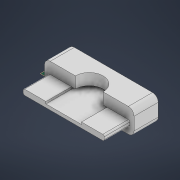
# Autodesk Inventor part: syringe_sledge_fitter
Saved by Autodesk Inventor 2022 (Build 260153000, 153)
## iProperties
Created: 2023-04-24
Part Number: syringe_sledge_fitter
Material: Generic
Document SubType Name: Modeling
Designer: Jakob Saugbjerg
Density: 1 g/cm^3
Appearance: Default
Author: Jakob Saugbjerg
Autodesk Inventor part; units mm, degrees
ref_plane "YZ Plane" through (0, 0, 0) normal (1, 0, 0) x (0, 1, 0)
ref_plane "XZ Plane" through (0, 0, 0) normal (0, 1, 0) x (-1, 0, 0)
ref_plane "XY Plane" through (0, 0, 0) normal (0, 0, 1) x (1, 0, 0)
sketch "Sketch1" plane through (0, 0, 0) normal (0, 0, 1) x (1, 0, 0)
  line L0 (0, 0) -> (63, 0)
  line L1 (63, 0) -> (63, 17)
  line L2 (63, 17) -> (0, 17)
  line L3 (0, 17) -> (0, 0)
  dimension "d0" = 63
  dimension "d1" = 17
  constraints: 8 end point, 2 parallel, 1 horizontal, 1 perpendicular
  measures "d0" distance of L2.end L1.end
  measures "d1" distance of L1.end L0.end
extrude "Extrusion1" add sketch "Sketch1" along normal blind 35
sketch "Sketch2" plane through (0, 17, 0) normal (0, 1, 0) x (1, 0, 0)
  line L0 (31.5, -35) -> (31.5, -17)
  circle A0 centre (31.5, -17) radius 9.75
  line L1 (63, -35) -> (0, -35) projected
  line L2 (21.75, -17) -> (41.25, -17)
  line L3 (41.25, -17) -> (41.25, -35)
  line L4 (41.25, -35) -> (21.75, -35)
  line L5 (21.75, -35) -> (21.75, -17)
  point P0 (0, 0)
  dimension "d37" = 19.5
  dimension "d36" = 18
  constraints: 10 end point, 2 parallel, 1 coincident, 1 horizontal, 1 perpendicular, 1 point on line, 1 vertical, 3 other
  measures "d36" distance of L0.start L0.end
extrude "20 mL cross" cut sketch "Sketch2" against normal blind 8
sketch "Sketch3" plane through (0, 9, 0) normal (0, 1, 0) x (1, 0, 0)
  arc A0 (41.25, -17) -> (21.75, -17) centre (31.5, -17) ccw projected
  circle A1 centre (31.5, -17) radius 12.5
  line L0 (19, -17) -> (44, -17)
  line L1 (44, -17) -> (44, -35)
  line L2 (44, -35) -> (19, -35)
  line L3 (19, -35) -> (19, -17)
  point P0 (0, 0)
  point P1 (41.1047, -25)
  dimension "d40" = 25
  constraints: 8 end point, 2 parallel, 2 point on circle, 1 centre point, 1 coincident, 1 horizontal, 1 perpendicular
  measures "d40" diameter of A1
extrude "20 mL top" cut sketch "Sketch3" against normal blind 1.5
sketch "Sketch4" plane through (0, 17, 0) normal (0, 1, 0) x (1, 0, 0)
  line L0 (63, -35) -> (0, -35)
  line L1 (0, -35) -> (0, -17)
  line L2 (0, -17) -> (63, -17)
  line L3 (63, -17) -> (63, -35)
  point P0 (0, 0)
  dimension "d19" = 63
  dimension "d20" = 18
  constraints: 8 end point, 2 parallel, 1 horizontal, 1 perpendicular
  measures "d19" distance of L1.end L2.end
  measures "d20" distance of L0.end L1.end
extrude "Extrusion4" cut sketch "Sketch4" against normal blind 8
sketch "Sketch10" plane through (0, 0, 0) normal (0, 0, -1) x (-1, 0, 0)
  line L0 (-19.9115, 8.8287) -> (-18.0318, 8.8287)
  line L1 (-18.0318, 8.8287) -> (-18.0318, 8.3965)
  spline S0 degree 2 poles (-18.0318, 8.3965) (-18.2344, 8.2063) (-18.595, 7.8531) (-18.7679, 7.6629) knots 0 0 0 1 2 2 2
  spline S1 degree 2 poles (-18.7679, 7.6629) (-19.1162, 7.28) (-19.3706, 6.8206) (-19.3706, 6.5761) knots 0 0 0 1 2 2 2
  spline S2 degree 2 poles (-19.3706, 6.5761) (-19.3706, 6.4476) (-19.2915, 6.255) (-19.2199, 6.1932) knots 0 0 0 1 2 2 2
  spline S3 degree 2 poles (-19.2199, 6.1932) (-19.1483, 6.1315) (-18.9606, 6.0697) (-18.8469, 6.0697) knots 0 0 0 1 2 2 2
  spline S4 degree 2 poles (-18.8469, 6.0697) (-18.7383, 6.0697) (-18.5159, 6.1241) (-18.4147, 6.1661) knots 0 0 0 1 2 2 2
  spline S5 degree 2 poles (-18.4147, 6.1661) (-18.3282, 6.2006) (-18.1677, 6.2994) (-18.1183, 6.334) knots 0 0 0 1 2 2 2
  line L2 (-18.1183, 6.334) -> (-18.096, 6.334)
  line L3 (-18.096, 6.334) -> (-18.096, 5.8993)
  spline S6 degree 2 poles (-18.096, 5.8993) (-18.222, 5.8375) (-18.674, 5.7165) (-18.8766, 5.7165) knots 0 0 0 1 2 2 2
  spline S7 degree 2 poles (-18.8766, 5.7165) (-19.3039, 5.7165) (-19.7855, 6.1685) (-19.7855, 6.5539) knots 0 0 0 1 2 2 2
  spline S8 degree 2 poles (-19.7855, 6.5539) (-19.7855, 6.7342) (-19.7016, 7.0355) (-19.6275, 7.1639) knots 0 0 0 1 2 2 2
  spline S9 degree 2 poles (-19.6275, 7.1639) (-19.5534, 7.2973) (-19.3385, 7.5591) (-19.2199, 7.6851) knots 0 0 0 1 2 2 2
  spline S10 degree 2 poles (-19.2199, 7.6851) (-19.0272, 7.8951) (-18.5555, 8.3446) (-18.4147, 8.4755) knots 0 0 0 1 2 2 2
  line L4 (-18.4147, 8.4755) -> (-19.9115, 8.4755)
  line L5 (-19.9115, 8.4755) -> (-19.9115, 8.8287)
  spline S11 degree 2 poles (-22.216, 7.3047) (-22.216, 8.1248) (-21.7393, 8.893) (-21.2428, 8.893) knots 0 0 0 1 2 2 2
  spline S12 degree 2 poles (-21.2428, 8.893) (-20.739, 8.893) (-20.2672, 8.11) (-20.2672, 7.3072) knots 0 0 0 1 2 2 2
  spline S13 degree 2 poles (-20.2672, 7.3072) (-20.2672, 6.4822) (-20.7439, 5.719) (-21.2428, 5.719) knots 0 0 0 1 2 2 2
  spline S14 degree 2 poles (-21.2428, 5.719) (-21.7443, 5.719) (-22.216, 6.5094) (-22.216, 7.3047) knots 0 0 0 1 2 2 2
  spline S15 degree 2 poles (-21.6924, 8.2335) (-21.7517, 8.0828) (-21.8011, 7.6184) (-21.8011, 7.3047) knots 0 0 0 1 2 2 2
  spline S16 degree 2 poles (-21.8011, 7.3047) (-21.8011, 6.991) (-21.7517, 6.5292) (-21.6899, 6.3735) knots 0 0 0 1 2 2 2
  spline S17 degree 2 poles (-21.6899, 6.3735) (-21.6282, 6.2179) (-21.4133, 6.0574) (-21.2428, 6.0574) knots 0 0 0 1 2 2 2
  spline S18 degree 2 poles (-21.2428, 6.0574) (-21.0724, 6.0574) (-20.8526, 6.2179) (-20.7884, 6.3785) knots 0 0 0 1 2 2 2
  spline S19 degree 2 poles (-20.7884, 6.3785) (-20.7266, 6.5341) (-20.6822, 7.0083) (-20.6822, 7.3072) knots 0 0 0 1 2 2 2
  spline S20 degree 2 poles (-20.6822, 7.3072) (-20.6822, 7.6283) (-20.7217, 8.0581) (-20.7859, 8.2261) knots 0 0 0 1 2 2 2
  spline S21 degree 2 poles (-20.7859, 8.2261) (-20.8452, 8.3841) (-21.065, 8.5546) (-21.2428, 8.5546) knots 0 0 0 1 2 2 2
  spline S22 degree 2 poles (-21.2428, 8.5546) (-21.4108, 8.5546) (-21.6306, 8.394) (-21.6924, 8.2335) knots 0 0 0 1 2 2 2
  line L6 (-26.5657, 8.8287) -> (-26.5657, 7.5048)
  spline S23 degree 2 poles (-26.5657, 7.5048) (-26.5657, 7.3467) (-26.541, 7.0775) (-26.5015, 7.0034) knots 0 0 0 1 2 2 2
  spline S24 degree 2 poles (-26.5015, 7.0034) (-26.462, 6.9219) (-26.3113, 6.8428) (-26.1804, 6.8428) knots 0 0 0 1 2 2 2
  spline S25 degree 2 poles (-26.1804, 6.8428) (-26.0618, 6.8428) (-25.7901, 6.9886) (-25.6469, 7.1269) knots 0 0 0 1 2 2 2
  spline S26 degree 2 poles (-25.6469, 7.1269) (-25.6494, 7.1615) (-25.6543, 7.2578) (-25.6543, 7.322) knots 0 0 0 1 2 2 2
  line L7 (-25.6543, 7.322) -> (-25.6543, 8.8287)
  line L8 (-25.6543, 8.8287) -> (-25.269, 8.8287)
  line L9 (-25.269, 8.8287) -> (-25.269, 7.5048)
  spline S27 degree 2 poles (-25.269, 7.5048) (-25.269, 7.3467) (-25.2443, 7.0775) (-25.2048, 7.0034) knots 0 0 0 1 2 2 2
  spline S28 degree 2 poles (-25.2048, 7.0034) (-25.1652, 6.9219) (-25.0146, 6.8428) (-24.8837, 6.8428) knots 0 0 0 1 2 2 2
  spline S29 degree 2 poles (-24.8837, 6.8428) (-24.7601, 6.8428) (-24.486, 6.9985) (-24.3575, 7.1195) knots 0 0 0 1 2 2 2
  line L10 (-24.3575, 7.1195) -> (-24.3575, 8.8287)
  line L11 (-24.3575, 8.8287) -> (-23.9722, 8.8287)
  line L12 (-23.9722, 8.8287) -> (-23.9722, 6.5415)
  line L13 (-23.9722, 6.5415) -> (-24.3575, 6.5415)
  line L14 (-24.3575, 6.5415) -> (-24.3575, 6.7934)
  spline S30 degree 2 poles (-24.3575, 6.7934) (-24.5082, 6.6428) (-24.8046, 6.4773) (-24.9825, 6.4773) knots 0 0 0 1 2 2 2
  spline S31 degree 2 poles (-24.9825, 6.4773) (-25.185, 6.4773) (-25.4987, 6.6625) (-25.5802, 6.8725) knots 0 0 0 1 2 2 2
  spline S32 degree 2 poles (-25.5802, 6.8725) (-25.7556, 6.6774) (-26.0865, 6.4773) (-26.2792, 6.4773) knots 0 0 0 1 2 2 2
  spline S33 degree 2 poles (-26.2792, 6.4773) (-26.4274, 6.4773) (-26.6695, 6.5687) (-26.7584, 6.6724) knots 0 0 0 1 2 2 2
  spline S34 degree 2 poles (-26.7584, 6.6724) (-26.8498, 6.7762) (-26.9511, 7.0874) (-26.9511, 7.322) knots 0 0 0 1 2 2 2
  line L15 (-26.9511, 7.322) -> (-26.9511, 8.8287)
  line L16 (-26.9511, 8.8287) -> (-26.5657, 8.8287)
  line L17 (-29.2877, 8.8287) -> (-27.5216, 8.8287)
  line L18 (-27.5216, 8.8287) -> (-27.5216, 5.7807)
  line L19 (-27.5216, 5.7807) -> (-27.9267, 5.7807)
  line L20 (-27.9267, 5.7807) -> (-27.9267, 8.4681)
  line L21 (-27.9267, 8.4681) -> (-29.2877, 8.4681)
  line L22 (-29.2877, 8.4681) -> (-29.2877, 8.8287)
  spline S35 degree 2 poles (-31.5033, 8.8831) (-31.2736, 8.8831) (-30.8759, 8.7596) (-30.745, 8.6904) knots 0 0 0 1 2 2 2
  line L23 (-30.745, 8.6904) -> (-30.745, 8.2582)
  line L24 (-30.745, 8.2582) -> (-30.7648, 8.2582)
  spline S36 degree 2 poles (-30.7648, 8.2582) (-30.8142, 8.2977) (-30.9475, 8.3915) (-31.0587, 8.4434) knots 0 0 0 1 2 2 2
  spline S37 degree 2 poles (-31.0587, 8.4434) (-31.155, 8.4903) (-31.3921, 8.5595) (-31.5181, 8.5595) knots 0 0 0 1 2 2 2
  spline S38 degree 2 poles (-31.5181, 8.5595) (-31.6095, 8.5595) (-31.8195, 8.5175) (-31.8689, 8.4829) knots 0 0 0 1 2 2 2
  spline S39 degree 2 poles (-31.8689, 8.4829) (-31.9405, 8.436) (-32.0047, 8.3298) (-32.0047, 8.2211) knots 0 0 0 1 2 2 2
  spline S40 degree 2 poles (-32.0047, 8.2211) (-32.0047, 8.0853) (-31.8565, 7.9445) (-31.6663, 7.8975) knots 0 0 0 1 2 2 2
  spline S41 degree 2 poles (-31.6663, 7.8975) (-31.5922, 7.8803) (-31.3551, 7.8309) (-31.2538, 7.8037) knots 0 0 0 1 2 2 2
  spline S42 degree 2 poles (-31.2538, 7.8037) (-30.992, 7.7271) (-30.7549, 7.4109) (-30.7549, 7.1862) knots 0 0 0 1 2 2 2
  spline S43 degree 2 poles (-30.7549, 7.1862) (-30.7549, 6.875) (-31.2217, 6.4872) (-31.607, 6.4872) knots 0 0 0 1 2 2 2
  spline S44 degree 2 poles (-31.607, 6.4872) (-31.7972, 6.4872) (-32.1825, 6.581) (-32.3135, 6.6527) knots 0 0 0 1 2 2 2
  line L25 (-32.3135, 6.6527) -> (-32.3135, 7.0651)
  line L26 (-32.3135, 7.0651) -> (-32.2937, 7.0651)
  spline S45 degree 2 poles (-32.2937, 7.0651) (-32.1455, 6.9466) (-31.7849, 6.8107) (-31.5996, 6.8107) knots 0 0 0 1 2 2 2
  spline S46 degree 2 poles (-31.5996, 6.8107) (-31.4094, 6.8107) (-31.1476, 6.9713) (-31.1476, 7.1318) knots 0 0 0 1 2 2 2
  spline S47 degree 2 poles (-31.1476, 7.1318) (-31.1476, 7.2776) (-31.3032, 7.4184) (-31.4761, 7.4628) knots 0 0 0 1 2 2 2
  spline S48 degree 2 poles (-31.4761, 7.4628) (-31.5601, 7.485) (-31.7725, 7.5295) (-31.8886, 7.5567) knots 0 0 0 1 2 2 2
  spline S49 degree 2 poles (-31.8886, 7.5567) (-32.1406, 7.6209) (-32.3974, 7.9148) (-32.3974, 8.1692) knots 0 0 0 1 2 2 2
  spline S50 degree 2 poles (-32.3974, 8.1692) (-32.3974, 8.3174) (-32.2813, 8.5793) (-32.1677, 8.6756) knots 0 0 0 1 2 2 2
  spline S51 degree 2 poles (-32.1677, 8.6756) (-32.0467, 8.7769) (-31.7379, 8.8831) (-31.5033, 8.8831) knots 0 0 0 1 2 2 2
  line L27 (-34.5513, 6.5415) -> (-33.3212, 9.671)
  line L28 (-33.3212, 9.671) -> (-32.9087, 9.671)
  line L29 (-32.9087, 9.671) -> (-33.3188, 8.7176)
  line L30 (-33.3188, 8.7176) -> (-32.4888, 6.5415)
  line L31 (-32.4888, 6.5415) -> (-32.9038, 6.5415)
  line L32 (-32.9038, 6.5415) -> (-33.5287, 8.2359)
  line L33 (-33.5287, 8.2359) -> (-34.1512, 6.5415)
  line L34 (-34.1512, 6.5415) -> (-34.5513, 6.5415)
  line L35 (-36.0555, 6.954) -> (-36.0358, 6.954)
  spline S52 degree 2 poles (-36.0358, 6.954) (-35.9913, 6.9416) (-35.895, 6.9367) (-35.8283, 6.9367) knots 0 0 0 1 2 2 2
  spline S53 degree 2 poles (-35.8283, 6.9367) (-35.6727, 6.9367) (-35.3664, 7.0726) (-35.2281, 7.2059) knots 0 0 0 1 2 2 2
  line L36 (-35.2281, 7.2059) -> (-35.2281, 8.8287)
  line L37 (-35.2281, 8.8287) -> (-34.8428, 8.8287)
  line L38 (-34.8428, 8.8287) -> (-34.8428, 6.5415)
  line L39 (-34.8428, 6.5415) -> (-35.2281, 6.5415)
  line L40 (-35.2281, 6.5415) -> (-35.2281, 6.8824)
  spline S54 degree 2 poles (-35.2281, 6.8824) (-35.438, 6.6946) (-35.7517, 6.5415) (-35.8999, 6.5415) knots 0 0 0 1 2 2 2
  spline S55 degree 2 poles (-35.8999, 6.5415) (-35.9592, 6.5415) (-36.0185, 6.5464) (-36.0555, 6.5539) knots 0 0 0 1 2 2 2
  line L41 (-36.0555, 6.5539) -> (-36.0555, 6.954)
  line L42 (-36.7471, 8.8287) -> (-36.3618, 8.8287)
  line L43 (-36.3618, 8.8287) -> (-36.3618, 6.5415)
  line L44 (-36.3618, 6.5415) -> (-36.7471, 6.5415)
  line L45 (-36.7471, 6.5415) -> (-36.7471, 8.8287)
  line L46 (-36.7743, 6.1611) -> (-36.3371, 6.1611)
  line L47 (-36.3371, 6.1611) -> (-36.3371, 5.761)
  line L48 (-36.3371, 5.761) -> (-36.7743, 5.761)
  line L49 (-36.7743, 5.761) -> (-36.7743, 6.1611)
  line L50 (-39.1085, 8.8287) -> (-38.7232, 8.8287)
  line L51 (-38.7232, 8.8287) -> (-38.7232, 7.5246)
  spline S56 degree 2 poles (-38.7232, 7.5246) (-38.7232, 7.3665) (-38.6935, 7.0948) (-38.6491, 7.0133) knots 0 0 0 1 2 2 2
  spline S57 degree 2 poles (-38.6491, 7.0133) (-38.6021, 6.9268) (-38.4342, 6.8428) (-38.2909, 6.8428) knots 0 0 0 1 2 2 2
  spline S58 degree 2 poles (-38.2909, 6.8428) (-38.1476, 6.8428) (-37.8438, 6.996) (-37.6981, 7.1195) knots 0 0 0 1 2 2 2
  line L52 (-37.6981, 7.1195) -> (-37.6981, 8.8287)
  line L53 (-37.6981, 8.8287) -> (-37.3128, 8.8287)
  line L54 (-37.3128, 8.8287) -> (-37.3128, 6.5415)
  line L55 (-37.3128, 6.5415) -> (-37.6981, 6.5415)
  line L56 (-37.6981, 6.5415) -> (-37.6981, 6.7959)
  spline S59 degree 2 poles (-37.6981, 6.7959) (-37.871, 6.6403) (-38.2044, 6.4773) (-38.3922, 6.4773) knots 0 0 0 1 2 2 2
  spline S60 degree 2 poles (-38.3922, 6.4773) (-38.7281, 6.4773) (-39.1085, 6.9219) (-39.1085, 7.3443) knots 0 0 0 1 2 2 2
  line L57 (-39.1085, 7.3443) -> (-39.1085, 8.8287)
  spline S61 degree 2 poles (-39.7309, 9.1943) (-39.7704, 9.2116) (-39.9211, 9.2659) (-40.0174, 9.2882) knots 0 0 0 1 2 2 2
  spline S62 degree 2 poles (-40.0174, 9.2882) (-40.1237, 9.3153) (-40.304, 9.3474) (-40.4102, 9.3474) knots 0 0 0 1 2 2 2
  spline S63 degree 2 poles (-40.4102, 9.3474) (-40.588, 9.3474) (-40.835, 9.2536) (-40.9042, 9.1696) knots 0 0 0 1 2 2 2
  spline S64 degree 2 poles (-40.9042, 9.1696) (-40.9709, 9.0856) (-41.0227, 8.8658) (-41.0227, 8.725) knots 0 0 0 1 2 2 2
  line L58 (-41.0227, 8.725) -> (-41.0227, 8.5249)
  spline S65 degree 2 poles (-41.0227, 8.5249) (-40.8671, 8.6608) (-40.5683, 8.7892) (-40.3435, 8.7892) knots 0 0 0 1 2 2 2
  spline S66 degree 2 poles (-40.3435, 8.7892) (-39.9532, 8.7892) (-39.4913, 8.2088) (-39.4913, 7.6629) knots 0 0 0 1 2 2 2
  spline S67 degree 2 poles (-39.4913, 7.6629) (-39.4913, 7.3788) (-39.6519, 6.9392) (-39.7853, 6.7836) knots 0 0 0 1 2 2 2
  spline S68 degree 2 poles (-39.7853, 6.7836) (-39.9137, 6.6378) (-40.2669, 6.4773) (-40.4546, 6.4773) knots 0 0 0 1 2 2 2
  spline S69 degree 2 poles (-40.4546, 6.4773) (-40.6325, 6.4773) (-40.8918, 6.5613) (-41.0227, 6.6378) knots 0 0 0 1 2 2 2
  line L59 (-41.0227, 6.6378) -> (-41.045, 6.5415)
  line L60 (-41.045, 6.5415) -> (-41.4081, 6.5415)
  line L61 (-41.4081, 6.5415) -> (-41.4081, 8.5669)
  spline S70 degree 2 poles (-41.4081, 8.5669) (-41.4081, 9.1498) (-40.9017, 9.6932) (-40.3805, 9.6932) knots 0 0 0 1 2 2 2
  spline S71 degree 2 poles (-40.3805, 9.6932) (-40.2126, 9.6932) (-39.8618, 9.6389) (-39.7112, 9.5944) knots 0 0 0 1 2 2 2
  line L62 (-39.7112, 9.5944) -> (-39.7112, 9.1943)
  line L63 (-39.7112, 9.1943) -> (-39.7309, 9.1943)
  line L64 (-41.0227, 8.2088) -> (-41.0227, 6.9515)
  spline S72 degree 2 poles (-41.0227, 6.9515) (-40.8795, 6.8824) (-40.6374, 6.8231) (-40.5164, 6.8231) knots 0 0 0 1 2 2 2
  spline S73 degree 2 poles (-40.5164, 6.8231) (-40.2249, 6.8231) (-39.889, 7.2529) (-39.889, 7.6555) knots 0 0 0 1 2 2 2
  spline S74 degree 2 poles (-39.889, 7.6555) (-39.889, 8.0359) (-40.1434, 8.4335) (-40.4299, 8.4335) knots 0 0 0 1 2 2 2
  spline S75 degree 2 poles (-40.4299, 8.4335) (-40.5806, 8.4335) (-40.8968, 8.315) (-41.0227, 8.2088) knots 0 0 0 1 2 2 2
  spline S76 degree 2 poles (-42.9592, 8.8806) (-42.4109, 8.8806) (-41.8082, 8.2656) (-41.8082, 7.6975) knots 0 0 0 1 2 2 2
  spline S77 degree 2 poles (-41.8082, 7.6975) (-41.8082, 7.1392) (-42.3936, 6.4773) (-42.8654, 6.4773) knots 0 0 0 1 2 2 2
  spline S78 degree 2 poles (-42.8654, 6.4773) (-43.0778, 6.4773) (-43.4063, 6.6008) (-43.5273, 6.7317) knots 0 0 0 1 2 2 2
  spline S79 degree 2 poles (-43.5273, 6.7317) (-43.6508, 6.8626) (-43.7817, 7.2405) (-43.7817, 7.5147) knots 0 0 0 1 2 2 2
  line L65 (-43.7817, 7.5147) -> (-43.7817, 7.7246)
  line L66 (-43.7817, 7.7246) -> (-42.1985, 7.7246)
  spline S80 degree 2 poles (-42.1985, 7.7246) (-42.1985, 8.1223) (-42.5986, 8.5447) (-42.9543, 8.5447) knots 0 0 0 1 2 2 2
  spline S81 degree 2 poles (-42.9543, 8.5447) (-43.0803, 8.5447) (-43.3248, 8.4879) (-43.4236, 8.4434) knots 0 0 0 1 2 2 2
  spline S82 degree 2 poles (-43.4236, 8.4434) (-43.5273, 8.394) (-43.6706, 8.3076) (-43.7175, 8.268) knots 0 0 0 1 2 2 2
  line L67 (-43.7175, 8.268) -> (-43.7398, 8.268)
  line L68 (-43.7398, 8.268) -> (-43.7398, 8.6879)
  spline S83 degree 2 poles (-43.7398, 8.6879) (-43.6731, 8.7151) (-43.4705, 8.7942) (-43.3915, 8.8164) knots 0 0 0 1 2 2 2
  spline S84 degree 2 poles (-43.3915, 8.8164) (-43.2803, 8.8485) (-43.0976, 8.8806) (-42.9592, 8.8806) knots 0 0 0 1 2 2 2
  spline S85 degree 2 poles (-43.4063, 7.4307) (-43.4014, 7.2751) (-43.3371, 7.0479) (-43.2754, 6.9713) knots 0 0 0 1 2 2 2
  spline S86 degree 2 poles (-43.2754, 6.9713) (-43.2087, 6.8848) (-42.9987, 6.7934) (-42.8431, 6.7934) knots 0 0 0 1 2 2 2
  spline S87 degree 2 poles (-42.8431, 6.7934) (-42.69, 6.7934) (-42.4751, 6.8848) (-42.3862, 6.9738) knots 0 0 0 1 2 2 2
  spline S88 degree 2 poles (-42.3862, 6.9738) (-42.2997, 7.0651) (-42.2108, 7.285) (-42.1985, 7.4307) knots 0 0 0 1 2 2 2
  line L69 (-42.1985, 7.4307) -> (-43.4063, 7.4307)
  point P0 (0, 0)
  point P1 (-17.8095, 5.7165)
  dimension "d3" = 0
  constraints: 1 other
emboss "Emboss1" sketch "Sketch10" operation cut depth 1 direction (0, 0, 1)
ref_plane "Work Plane1" through (2, 0, 0) normal (0, -1, 0) x (1, 0, 0)
sketch "Sketch11" plane through (2, 0, 0) normal (0, -1, 0) x (1, 0, 0)
  line L0 (-2, 35) -> (-2, 0) projected
  line L1 (61, 17) -> (61, 35) projected
  line L2 (-2, 35) -> (61, 35)
  line L3 (61, 35) -> (61, 17)
  line L4 (61, 17) -> (-2, 17)
  line L5 (-2, 17) -> (-2, 35)
  point P0 (-2, 17)
  dimension "d41" = 18
  constraints: 8 end point, 2 parallel, 1 horizontal, 1 perpendicular
  measures "d41" distance of L2.end L1.start
extrude "Extrusion8" cut sketch "Sketch11" against normal blind 5.2
sketch "Sketch13" plane through (0, 0, 35) normal (0, 0, 1) x (1, 0, 0)
  line L0 (63, 3.2) -> (0, 3.2) projected
  line L1 (0, 9) -> (63, 9) projected
  line L2 (0, 3.2) -> (3, 3.2)
  line L3 (3, 3.2) -> (3, 9)
  line L4 (3, 9) -> (0, 9)
  line L5 (0, 9) -> (0, 3.2)
  line L6 (63, 9) -> (0, 9) projected
  line L7 (63, 9) -> (60, 9)
  line L8 (60, 9) -> (60, 3.2)
  line L9 (60, 3.2) -> (63, 3.2)
  line L10 (63, 3.2) -> (63, 9)
  point P0 (0, 0)
  point P1 (0, 9)
  point P2 (19, 7)
  point P3 (41.1047, 7)
  point P4 (60, 9)
  point P5 (60, 3.2)
  point P6 (0, 9)
  dimension "d52" = 3
  dimension "d53" = 3
  constraints: 16 end point, 4 parallel, 2 horizontal, 2 perpendicular, 1 point on line, 3 other
  measures "d52" distance of L4.end L3.end
  measures "d53" distance of L9.end L8.end
extrude "Extrusion10" cut sketch "Sketch13" against normal blind 18 contours L0 L8 L1 L10 | L0 L5 L1 L3
fillet "Fillet5" radius 1 4 edges at (3, 9, 26) (60, 9, 26) (3, 5.2, 26) (60, 5.2, 26)
fillet "Fillet6" radius 4 4 edges at (63, 17, 8.5) (63, 0, 8.5) (0, 17, 8.5) (0, 0, 8.5)
body "Solid1"
